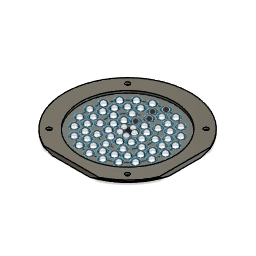
3.25 speaker grill-slice-off v1.0 (Autodesk Fusion 360 design; units mm, degrees)
Autodesk Fusion 360 part; units mm, degrees
sketch "Sketch1" plane through (0, 0, 0) normal (0, 1, 0) x (1, 0, 0)
  circle A0 centre (0, 0) radius 57.5
  line L0 (36, -36) -> (-36, -36) construction
  line L1 (-36, -36) -> (-36, 36) construction
  line L2 (-36, 36) -> (36, 36) construction
  line L3 (36, 36) -> (36, -36) construction
  line L4 (36, -36) -> (-36, 36) construction
  line L5 (-36, -36) -> (36, 36) construction
  circle A1 centre (0, 0) radius 43
  circle A2 centre (-36, 36) radius 2
  circle A3 centre (36, 36) radius 2
  circle A4 centre (36, -36) radius 2
  circle A5 centre (-36, -36) radius 2
  circle A6 centre (-36, -36) radius 2.875
  circle A7 centre (36, -36) radius 2.875
  circle A8 centre (36, 36) radius 2.875
  circle A9 centre (-36, 36) radius 2.875
  line L6 (52.5, 40.4773) -> (52.5, -51.7956) construction
  line L7 (67.5556, 30.3847) -> (52.5, 30.3847)
  line L8 (52.5, 30.3847) -> (52.5, -29.8632)
  line L9 (-46.2969, -51.75) -> (48.3967, -51.75)
  arc A10 (-25.0637, -51.75) -> (25.0637, -51.75) centre (0, 0) ccw
  dimension "d1" = 115
  dimension "d2" = 72
  dimension "d3" = 72
  dimension "d4" = 86
  dimension "d5" = 4
  dimension "d6" = 4
  dimension "d7" = 4
  dimension "d8" = 4
  dimension "d9" = 5.75
  dimension "d10" = 5.75
  dimension "d11" = 5.75
  dimension "d12" = 5.75
  dimension "d54" = 52.5
  dimension "d58" = 51.75
  constraint coincident A0.centre A1.centre
  constraint horizontal L0
  constraint perpendicular L0 L1
  constraint parallel L0 L2
  constraint parallel L1 L3
  constraint coincident L4 A0.centre
  constraint coincident L5 A0.centre
  constraint concentric A0 A1
  constraint coincident L1.end L2.start
  constraint coincident L2.end L3.start
  constraint coincident L0.start L3.end
  constraint coincident L0.end L1.start
  constraint concentric A5 A6
  constraint concentric A4 A7
  constraint concentric A3 A8
  constraint concentric A2 A9
  constraint vertical L6
  constraint horizontal L7
  constraint vertical L8
  constraint coincident L6 L8.end
  constraint horizontal L9
  constraint coincident A0 A10.end
  constraint coincident L9 A10.end
  constraint coincident A0 A10.start
  constraint coincident L9 A10.start
  measures "d1" diameter of A0
  measures "d2" distance of L1.end L2.end
  measures "d3" distance of L0.end L1.end
  measures "d4" diameter of A1
  measures "d5" diameter of A2
  measures "d6" diameter of A3
  measures "d7" diameter of A4
  measures "d8" diameter of A5
  measures "d9" diameter of A6
  measures "d10" diameter of A7
  measures "d11" diameter of A8
  measures "d12" diameter of A9
  measures "d54" distance of A0.centre L6
  measures "d58" distance of A0.centre L9
extrude "Extrude1" add sketch "Sketch1" along normal blind 4 contours A0 L9 A10 | A0 L8 L9 | A0 L8
extrude "Extrude3" add sketch "Sketch1" along normal blind 2 contours A1
sketch "Sketch2" plane through (0, 2, 0) normal (0, 1, 0) x (-1, 0, 0)
  circle A0 centre (0, 0) radius 43
  circle A1 centre (0, 0) radius 35 construction
  circle A2 centre (0, 0) radius 27.5 construction
  circle A3 centre (0, 0) radius 20 construction
  circle A4 centre (0, 0) radius 12.5 construction
  circle A5 centre (0, 0) radius 7.5 construction
  circle A6 centre (-0.2536, -34.9991) radius 3.5
  circle A7 centre (10.5741, -33.3645) radius 3.5
  circle A8 centre (20.3668, -28.4639) radius 3.5
  circle A9 centre (28.1658, -20.7771) radius 3.5
  circle A10 centre (33.2077, -11.0565) radius 3.5
  circle A11 centre (34.9991, -0.2536) radius 3.5
  circle A12 centre (33.3645, 10.5741) radius 3.5
  circle A13 centre (28.4639, 20.3668) radius 3.5
  circle A14 centre (20.7771, 28.1658) radius 3.5
  circle A15 centre (11.0565, 33.2077) radius 3.5
  circle A16 centre (0.2536, 34.9991) radius 3.5
  circle A17 centre (-10.5741, 33.3645) radius 3.5
  circle A18 centre (-20.3668, 28.4639) radius 3.5
  circle A19 centre (-28.1658, 20.7771) radius 3.5
  circle A20 centre (-33.2077, 11.0565) radius 3.5
  circle A21 centre (-34.9991, 0.2536) radius 3.5
  circle A22 centre (-33.3645, -10.5741) radius 3.5
  circle A23 centre (-28.4639, -20.3668) radius 3.5
  circle A24 centre (-20.7771, -28.1658) radius 3.5
  circle A25 centre (-11.0565, -33.2077) radius 3.5
  circle A26 centre (4.2963, -27.1623) radius 3.5
  circle A27 centre (12.4797, -24.5053) radius 3.5
  circle A28 centre (19.4414, -19.4495) radius 3.5
  circle A29 centre (24.5001, -12.4898) radius 3.5
  circle A30 centre (27.1605, -4.3076) radius 3.5
  circle A31 centre (27.1623, 4.2963) radius 3.5
  circle A32 centre (24.5053, 12.4797) radius 3.5
  circle A33 centre (19.4495, 19.4414) radius 3.5
  circle A34 centre (12.4898, 24.5001) radius 3.5
  circle A35 centre (4.3076, 27.1605) radius 3.5
  circle A36 centre (-4.2963, 27.1623) radius 3.5
  circle A37 centre (-12.4797, 24.5053) radius 3.5
  circle A38 centre (-19.4414, 19.4495) radius 3.5
  circle A39 centre (-24.5001, 12.4898) radius 3.5
  circle A40 centre (-27.1605, 4.3076) radius 3.5
  circle A41 centre (-27.1623, -4.2963) radius 3.5
  circle A42 centre (-24.5053, -12.4797) radius 3.5
  circle A43 centre (-19.4495, -19.4414) radius 3.5
  circle A44 centre (-12.4898, -24.5001) radius 3.5
  circle A45 centre (-4.3076, -27.1605) radius 3.5
  circle A46 centre (0.1335, -19.9996) radius 3.5
  circle A47 centre (11.8634, -16.1015) radius 3.5
  circle A48 centre (19.0619, -6.0533) radius 3.5
  circle A49 centre (18.9795, 6.3071) radius 3.5
  circle A50 centre (11.6475, 16.2584) radius 3.5
  circle A51 centre (-0.1335, 19.9996) radius 3.5
  circle A52 centre (-11.8634, 16.1015) radius 3.5
  circle A53 centre (-19.0619, 6.0533) radius 3.5
  circle A54 centre (-18.9795, -6.3071) radius 3.5
  circle A55 centre (-11.6475, -16.2584) radius 3.5
  circle A56 centre (4.3124, -11.7326) radius 3.5
  circle A57 centre (10.3851, -6.957) radius 3.5
  circle A58 centre (12.4909, 0.4758) radius 3.5
  circle A59 centre (9.8257, 7.7269) radius 3.5
  circle A60 centre (3.4074, 12.0266) radius 3.5
  circle A61 centre (-4.3124, 11.7326) radius 3.5
  circle A62 centre (-10.3851, 6.957) radius 3.5
  circle A63 centre (-12.4909, -0.4758) radius 3.5
  circle A64 centre (-9.8257, -7.7269) radius 3.5
  circle A65 centre (-3.4074, -12.0266) radius 3.5
  circle A66 centre (-0.0342, -5.0724) radius 2.5
  circle A67 centre (4.8135, -1.6) radius 2.5
  circle A68 centre (3.0092, 4.0835) radius 2.5
  circle A69 centre (-2.9538, 4.1238) radius 2.5
  circle A70 centre (-4.8347, -1.5349) radius 2.5
  dimension "d19" = 70
  dimension "d20" = 55
  dimension "d21" = 40
  dimension "d22" = 25
  dimension "d23" = 15
  dimension "d24" = 7
  dimension "d28" = 360
  dimension "d29" = 7
  dimension "d31" = 360
  dimension "d32" = 7
  dimension "d34" = 360
  dimension "d35" = 7
  dimension "d43" = 360
  dimension "d45" = 5
  dimension "d47" = 360
  constraint concentric A0 A1
  constraint concentric A1 A2
  constraint concentric A2 A3
  constraint concentric A2 A4
  constraint concentric A2 A5
  constraint coincident A1 A6.centre
  constraint coincident A2 A26.centre
  constraint coincident A3 A46.centre
  constraint coincident A4 A56.centre
  measures "d19" diameter of A1
  measures "d20" diameter of A2
  measures "d21" diameter of A3
  measures "d22" diameter of A4
  measures "d23" diameter of A5
  measures "d24" diameter of A6
  measures "d29" diameter of A26
  measures "d32" diameter of A46
  measures "d35" diameter of A56
  measures "d45" diameter of A66
extrude "Extrude4" cut sketch "Sketch2" against normal up to surface (2 mm away) contours A6
extrude "Extrude5" cut sketch "Sketch2" against normal up to surface (2 mm away) contours A7 | A8 | A9 | A10 | A11 | A12 | A13 | A14 | A15 | A16 | A17 | A18 | A19 | A20 | A21 | A22 | A23 | A24 | A25 | A26 | A27 | A28 | A29 | A30 | A31 | A32 | A33 | A34 | A35 | A36 | A37 | A38 | A39 | A40 | A41 | A42 | A43 | A44 | A45 | A46 | A47 | A48 | A49 | A50 | A51 | A52 | A53 | A54 | A55 | A56 | A57 | A58 | A59 | A60 | A61 | A62 | A63 | A64 | A65 | A66 | A67 | A68 | A69 | A70
extrude "Extrude6" add sketch "Sketch1" against normal blind 2 from surface at 4 contours A6 | A7 | A8 | A9
chamfer "Chamfer1" distance 3 angle 45 1 edges at (-53.6088, 0, 20.7929)
extrude "Extrude7" cut sketch "Sketch1" along normal up to surface (4 mm away) contours A0 L8
extrude "Extrude8" cut sketch "Sketch1" along normal up to surface (4 mm away) contours A0 L9 A10
equation "d54 = ( d1 / 2 ) - 5 mm"
equation "d58 = ( d1 / 2 ) - 5.75 mm"
